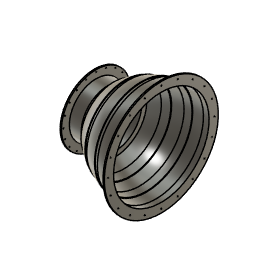
petrol_turbine_case_eng_model (Autodesk Fusion 360 design; units mm, degrees)
Autodesk Fusion 360 part; units mm, degrees
sketch "Sketch1" plane through (0, 0, 0) normal (0, 1, 0) x (1, 0, 0)
  line L0 (0, 0) -> (250.5, 0) construction
  line L1 (250.5, 0) -> (250.5, -213.77) construction
  line L2 (250.5, -213.77) -> (0, -213.77) construction
  line L3 (0, -213.77) -> (0, 0) construction
  dimension "d1" = 250.5
  dimension "d2" = 213.77
  constraint horizontal L0
  constraint vertical L1
  constraint horizontal L2
  constraint vertical L3
  constraint coincident L0.start L3.end
  measures "d1" distance of L0.start L0.end
  measures "d2" distance of L0.start L2.end
sketch "Sketch2" plane through (0, 0, 0) normal (0, 1, 0) x (1, 0, 0)
  line L0 (0, 0) -> (250, 0) construction
  line L1 (250, 0) -> (250, -129.65) construction
  line L2 (250, -129.65) -> (0, -129.65) construction
  line L3 (0, -129.65) -> (0, 0) construction
  line L4 (193.51, 174.3203) -> (193.51, 171.7713)
  line L5 (193.51, -171.7713) -> (193.51, -174.3361)
  line L6 (169.51, 168.436) -> (169.51, 165.8296)
  line L7 (169.51, -165.8296) -> (169.51, -168.436)
  line L8 (133.51, 155.0829) -> (133.51, 152.3361)
  line L9 (133.51, -152.3361) -> (133.51, -155.0829)
  line L10 (110.01, 143.0564) -> (110.01, 140.1696)
  line L11 (110.01, -140.1696) -> (110.01, -143.0564)
  line L12 (228.8785, 178.9674) -> (228.8785, -179.12)
  arc A0 (193.51, 171.7713) -> (169.51, 165.8296) centre (246.9617, -95.5777) ccw
  arc A1 (169.51, -165.8296) -> (193.51, -171.7713) centre (246.9617, 95.5777) ccw
  arc A2 (133.51, 152.3361) -> (110.01, 140.1696) centre (246.9617, -95.5777) ccw
  arc A3 (110.01, -140.1696) -> (133.51, -152.3361) centre (246.9617, 95.5777) ccw
  arc A4 (228.8785, 178.9674) -> (193.51, 174.3203) centre (246.9617, -95.5777) ccw
  arc A5 (193.51, -174.3361) -> (228.8785, -179.12) centre (247.9959, 95.355) ccw
  arc A6 (169.51, 168.436) -> (133.51, 155.0829) centre (246.9617, -95.5777) ccw
  arc A7 (133.51, -155.0829) -> (169.51, -168.436) centre (246.9617, 95.5777) ccw
  arc A8 (110.01, 143.0564) -> (75.51, 119.6114) centre (246.9617, -95.5777) ccw
  arc A9 (75.51, -119.6114) -> (110.01, -143.0564) centre (246.9617, 95.5777) ccw
  line L13 (0, -129.65) -> (0, -95)
  line L14 (0, -95) -> (50, -95)
  line L15 (334.2254, -100.76) -> (-102.5424, -100.76) construction
  line L16 (50, -95) -> (75.51, -100.76)
  line L17 (75.51, -100.76) -> (75.51, -119.6114)
  arc A10 (72.3943, -123.5219) -> (115.01, -151.54) centre (246.9617, 95.5777) ccw
  line L18 (115.01, -148.7023) -> (115.01, -151.54)
  arc A11 (115.01, -148.7023) -> (128.51, -155.5262) centre (246.9617, 95.5777) ccw
  line L19 (128.51, -155.5262) -> (128.51, -158.2876)
  arc A12 (128.51, -158.2876) -> (174.51, -175.0312) centre (246.9617, 95.5777) ccw
  line L20 (174.51, -172.4423) -> (174.51, -175.0312)
  arc A13 (174.51, -172.4423) -> (188.51, -175.8396) centre (246.9617, 95.5777) ccw
  line L21 (188.51, -175.8396) -> (188.51, -178.3964)
  arc A14 (188.51, -178.3964) -> (228.8785, -184.1319) centre (247.9959, 95.355) ccw
  line L22 (75.51, 119.6114) -> (75.51, 0)
  line L23 (75.51, -100.76) -> (75.51, -119.6114)
  line L24 (5, -129.65) -> (5, -100)
  line L25 (5, -100) -> (49.4425, -100)
  line L26 (49.4425, -100) -> (70.51, -104.7569)
  line L27 (70.51, -104.7569) -> (70.51, -122.0073)
  arc A15 (70.51, -122.0073) -> (107.5212, -147.393) centre (246.9617, 95.5777) ccw
  line L28 (5, -129.65) -> (0, -129.65)
  line L29 (250, 0) -> (250, -213.77) construction
  line L30 (228.8785, -184.1319) -> (245, -184.1319)
  line L31 (228.8785, -179.12) -> (250, -179.12)
  line L32 (250, -179.12) -> (250, -213.77)
  line L33 (250, -213.77) -> (245, -213.77)
  line L34 (245, -213.77) -> (245, -184.1319)
  dimension "d3" = 250
  dimension "d5" = 95
  dimension "d6" = 34.65
  dimension "d7" = 50
  dimension "d8" = 100.76
  dimension "d10" = 5
  dimension "d11" = 213.77
  dimension "d12" = 34.65
  dimension "d13" = 5
  constraint horizontal L0
  constraint vertical L1
  constraint horizontal L2
  constraint vertical L3
  constraint coincident L0.start L3.end
  constraint coincident L3 L13.end
  constraint perpendicular L3 L14
  constraint horizontal L15
  constraint coincident L15 L16.end
  constraint coincident L16.end L22
  constraint perpendicular L15 L17
  constraint concentric A9 A10
  constraint concentric A3 A11
  constraint concentric A7 A12
  constraint concentric A1 A13
  constraint concentric A5 A14
  constraint coincident L0 L22.end
  constraint collinear L22 L23
  constraint perpendicular L13 L28
  constraint perpendicular L0 L29
  constraint perpendicular L12 L31
  constraint coincident L29 L31.end
  constraint perpendicular L31 L32
  constraint perpendicular L29 L33
  constraint perpendicular L31 L34
  measures "d3" distance of L0.start L0.end
  measures "d5" distance of L0.start L13.end
  measures "d6" distance of L2.end L13.end
  measures "d7" distance of L13.end L14.end
  measures "d8" distance of L0.start L15
  measures "d11" distance of L0.end L29.end
  measures "d12" distance of L29.end L31.end
  measures "d13" distance of L29.end L33.end
revolve "Revolve1" add sketch "Sketch2" angle 360 about axis through (0, 0, 0) along (1, 0, 0)
sketch "Sketch3" plane through (0, 0, 0) normal (-1, 0, 0) x (0, -1, 0)
  circle A0 centre (0, 0) radius 129.65
  circle A1 centre (0, 0) radius 95
  line L0 (0, 0) -> (0, 238.1299) construction
  circle A2 centre (0, 122.5) radius 2
  dimension "d15" = 4
  dimension "d16" = 122.5
  constraint coincident A0.centre A1.centre
  constraint vertical L0
  constraint coincident L0 A2.centre
  measures "d15" diameter of A2
  measures "d16" distance of A0.centre A2.centre
extrude "Extrude1" cut sketch "Sketch3" against normal blind 35 contours A2
sketch "Sketch4" plane through (250, 0, 0) normal (1, 0, 0) x (0, 1, 0)
  circle A0 centre (0, 0) radius 179.12
  circle A1 centre (0, 0) radius 213.77
  line L0 (0, 0) -> (0, 246.5899) construction
  circle A2 centre (0, 200) radius 2
  dimension "d19" = 4
  dimension "d20" = 200
  constraint coincident A0.centre A1.centre
  constraint vertical L0
  constraint coincident L0 A2.centre
  measures "d19" diameter of A2
  measures "d20" distance of A0.centre A2.centre
extrude "Extrude2" cut sketch "Sketch4" against normal blind 27 contours A2
pattern_circular "C-Pattern1" count 20 over 360 about axis through (1.75, 0, 0) along (1, 0, 0) of "Extrude1", "Extrude2"
equation "d5 = ( 190 / 2 ) * 1 mm"
